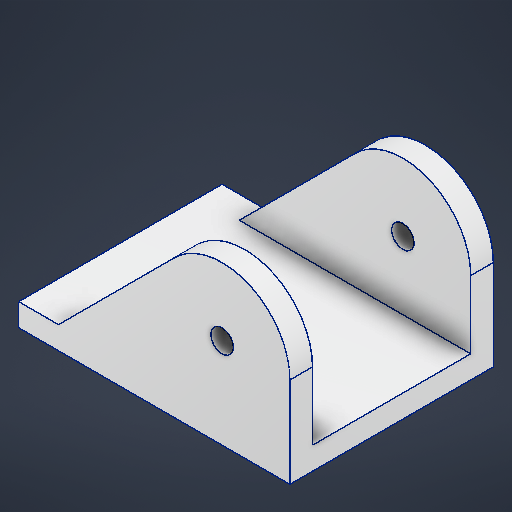
# Autodesk Inventor part: Foot
Saved by Autodesk Inventor 2026 (Build 300175000, 175)
## iProperties
Created: 2025-11-07
Part Number: Foot
Material: Aluminum 6061
Document SubType Name: Modeling
Designer: Study
Density: 2.7 g/cm^3
Appearance: Aluminum - Flat
Mass: 510.421 g
Surface Area: 440.513 cm^2
Volume: 189.045 cm^3
Author: Study
Autodesk Inventor part; units mm, degrees
ref_plane "YZ Plane" through (0, 0, 0) normal (1, 0, 0) x (0, 1, 0)
ref_plane "XZ Plane" through (0, 0, 0) normal (0, 1, 0) x (-1, 0, 0)
ref_plane "XY Plane" through (0, 0, 0) normal (0, 0, 1) x (1, 0, 0)
sketch "Sketch1" plane through (0, 0, 0) normal (0, 1, 0) x (-1, 0, 0)
  line L0 (0, 0) -> (-120, 0)
  line L1 (-120, 0) -> (-120, -90)
  line L2 (-120, -90) -> (0, -90)
  line L3 (0, -90) -> (0, 0)
  dimension "d0" = 120
  dimension "d1" = 90
  constraints: 8 end point, 2 parallel, 1 horizontal, 1 perpendicular
  measures "d0" distance of L2.end L1.end
  measures "d1" distance of L0.end L1.end
extrude "Extrusion1" add sketch "Sketch1" along normal blind 10
sketch "Sketch2" plane through (0, 10, 0) normal (0, 1, 0) x (1, 0, 0)
  point P0 (0, 0)
sketch "Sketch3" plane through (0, 10, 0) normal (0, 1, 0) x (1, 0, 0)
  line L0 (120, 0) -> (120, 90) projected
  line L1 (120, 0) -> (120, 10)
  line L2 (120, 10) -> (60, 10)
  line L3 (0, 0) -> (120, 0) projected
  line L4 (60, 10) -> (60, 0)
  line L5 (60, 0) -> (120, 0)
  line L6 (60, 0) -> (60, 90) construction
  line L7 (60, 90) -> (60, 80)
  line L8 (60, 80) -> (120, 80)
  line L9 (60, 90) -> (120, 90)
  line L10 (120, 90) -> (120, 80)
  dimension "d4" = 10
  dimension "d5" = 60
  dimension "d6" = 10
  constraints: 18 end point, 4 point on line, 2 collinear, 2 horizontal, 1 midpoint, 1 perpendicular
  measures "d4" distance of L0.start L1.end
  measures "d5" distance of L1.end L2.end
  measures "d6" distance of L6.end L7.end
extrude "Extrusion2" add sketch "Sketch3" along normal blind 60
sketch "Sketch4" plane through (0, 0, 0) normal (0, 0, 1) x (1, 0, 0)
  line L0 (60, 10) -> (60, 70) projected
  line L1 (120, 0) -> (120, 70) projected
  line L2 (60, 70) -> (120, 70)
  line L3 (120, 70) -> (120, 20)
  line L4 (120, 20) -> (60, 20)
  line L5 (60, 20) -> (60, 70)
  circle A0 centre (90, 40) radius 30
  circle A1 centre (90, 40) radius 5
  line L6 (67.8284, 60.2094) -> (135.2299, 60.2094) construction
  line L7 (67.8284, 60.2094) -> (17.619, 10)
  line L8 (60, 10) -> (0, 10) projected
  line L9 (67.8284, 60.2094) -> (138.8353, 60.2094) construction
  line L10 (120, 10) -> (60, 10) projected
  line L11 (17.619, 10) -> (60, 10)
  line L12 (60, 10) -> (60, 40)
  point P0 (0, 0)
  point P1 (90, 70)
  point P2 (120, 40)
  dimension "d9" = 50
  dimension "d10" = 10
  dimension "d14" = 135
  constraints: 18 end point, 3 horizontal, 3 point on line, 3 tangent, 2 centre point, 2 parallel, 2 point on circle, 1 coincident, 1 collinear, 1 equal length, 1 perpendicular
  measures "d9" distance of L2.end L3.end
  measures "d10" diameter of A1
  measures "d14" angle of L7 L9
extrude "Extrusion3" cut sketch "Sketch4" against normal blind 100 contours L0 L7 A0 | L0 L2 A0 L7 | A0 L2 L1 | A1
extrude "Extrusion4" add sketch "Sketch4" against normal blind 90 contours L8 L7 L0 | L0 L7 A0
sketch "Sketch5" plane through (0, 0, 0) normal (1, 0, 0) x (0, 1, 0)
  line L0 (10, -10) -> (40, -10) projected
  line L1 (10, -10) -> (10, -80) projected
  line L2 (10, -10) -> (10, -80)
  line L3 (10, -80) -> (63.3463, -80)
  line L4 (63.3463, -80) -> (63.3463, -10)
  line L5 (63.3463, -10) -> (10, -10)
  point P0 (0, 0)
  dimension "d19" = 70
  constraints: 8 end point, 3 equal length, 1 perpendicular
  measures "d19" distance of L3.end L4.end
extrude "Extrusion5" cut sketch "Sketch5" along normal blind 90
body "Solid1"
